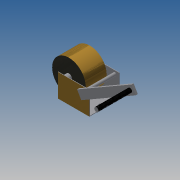
# Autodesk Inventor part: winch
Saved by Autodesk Inventor 2013 SP2 (Build 170200200, 200)
## iProperties
Created: 2013-12-16
Part Number: winch
Material: Generic
Document SubType Name: Modeling
Designer: Dave
Density: 1 g/cm^3
Author: Dave
Autodesk Inventor part; units mm, degrees
ref_plane "YZ Plane" through (0, 0, 0) normal (1, 0, 0) x (0, 1, 0)
ref_plane "XZ Plane" through (0, 0, 0) normal (0, 1, 0) x (-1, 0, 0)
ref_plane "XY Plane" through (0, 0, 0) normal (0, 0, 1) x (1, 0, 0)
sketch "Sketch1" plane through (0, 0, 0) normal (0, 0, 1) x (1, 0, 0)
  circle A0 centre (0, 0) radius 50.8
  dimension "d0" = 101.6
  constraints: 1 centre point, 1 coincident
  measures "d0" diameter of A0
extrude "Extrusion1" add sketch "Sketch1" along normal blind 63.5
sketch "Sketch2" plane through (0, 0, 63.5) normal (0, 0, 1) x (1, 0, 0)
  circle A0 centre (0, 0) radius 50.8 projected
  circle A1 centre (0, 0) radius 9.525
  dimension "d5" = 19.05
  constraints: 1 centre point, 1 coincident
  measures "d5" diameter of A1
extrude "Extrusion2" add sketch "Sketch2" along normal blind 15.875 and the other way blind 76.2 contours A1
sketch "Sketch3" plane through (0, 0, 79.375) normal (0, 0, 1) x (1, 0, 0)
  line L0 (-15.875, -55.5625) -> (79.375, -55.5625)
  line L1 (79.375, -55.5625) -> (79.375, 14.2875)
  line L2 (79.375, 14.2875) -> (-15.875, 14.2875)
  line L3 (-15.875, 14.2875) -> (-15.875, -55.5625)
  dimension "d11" = 95.25
  dimension "d13" = 69.85
  constraints: 8 end point, 2 parallel, 1 horizontal, 1 perpendicular
  measures "d11" distance of L0.start L0.end
  measures "d13" distance of L2.end L0.start
extrude "Extrusion3" add sketch "Sketch3" along normal blind 1.524
sketch "Sketch4" plane through (0, 0, 79.375) normal (0, 0, -1) x (-1, 0, 0)
  line L0 (15.875, -55.5625) -> (-79.375, -55.5625) projected
  line L1 (15.875, 14.2875) -> (15.875, -55.5625) projected
  line L2 (-79.375, -55.5625) -> (15.875, -55.5625)
  line L3 (15.875, -55.5625) -> (15.875, -54.0385)
  line L4 (15.875, -54.0385) -> (-79.375, -54.0385)
  line L5 (-79.375, -54.0385) -> (-79.375, -55.5625)
  point P0 (-79.375, 14.2875)
  dimension "d16" = 1.524
  dimension "d47" = 69.85
  dimension "d48" = 95.25
  constraints: 8 end point, 2 parallel, 1 horizontal, 1 perpendicular, 1 point on line
  measures "d16" distance of L4.end L0.end
  measures "d47" distance of L0.end point (-79.375, 14.288)
  measures "d48" distance of point (-79.375, 14.288) L1.start
extrude "Extrusion4" add sketch "Sketch4" along normal blind 88.9
sketch "Sketch5" plane through (0, 0, -9.525) normal (0, 0, -1) x (-1, 0, 0)
  line L0 (-79.375, -55.5625) -> (15.875, -55.5625)
  line L1 (15.875, -55.5625) -> (15.875, 14.2875)
  line L2 (15.875, 14.2875) -> (-79.375, 14.2875)
  line L3 (-79.375, 14.2875) -> (-79.375, -55.5625)
  point P0 (0, 0)
  constraints: 8 end point, 2 parallel, 1 horizontal, 1 perpendicular
extrude "Extrusion5" add sketch "Sketch5" along normal blind 1.524
sketch "Sketch6" plane through (0, 0, 80.899) normal (0, 0, 1) x (1, 0, 0)
  circle A0 centre (66.2655, 4.5181) radius 4.7625
  point P0 (0, 0)
  dimension "d21" = 9.525
  constraints: 1 centre point
  measures "d21" diameter of A0
extrude "Extrusion6" add sketch "Sketch6" along normal blind 12.7 and the other way blind 95.25
sketch "Sketch7" plane through (66.2655, 4.5181, 93.599) normal (0, 0, 1) x (1, 0, 0)
  line L0 (-5.1033, 11.8715) -> (159.8746, 107.1215)
  line L1 (159.8746, 107.1215) -> (172.5746, 85.1244)
  line L2 (172.5746, 85.1244) -> (7.5967, -10.1256)
  line L3 (7.5967, -10.1256) -> (-5.1033, 11.8715)
  line L4 (0, 0) -> (168.275, 0) construction
  point P0 (-66.2655, -4.5181)
  dimension "d29" = 25.4
  dimension "d30" = 190.5
  dimension "d40" = 30
  constraints: 10 end point, 2 parallel, 1 horizontal, 1 perpendicular
  measures "d29" distance of L2.end L0.start
  measures "d30" distance of L1.end L2.end
  measures "d40" angle of L4 L2
extrude "Extrusion7" add sketch "Sketch7" along normal blind 6.35
sketch "Sketch8" plane through (66.2655, 4.5181, 99.949) normal (0, 0, 1) x (1, 0, 0)
  line L0 (172.5746, 85.1244) -> (159.8746, 107.1215) projected
  circle A0 centre (155.226, 89.773) radius 6.35
  point P0 (-66.2655, -4.5181)
  dimension "d43" = 12.7
  dimension "d44" = 12.7
  constraints: 1 centre point
  measures "d43" diameter of A0
  measures "d44" distance from line of A0.centre L0
extrude "Extrusion8" add sketch "Sketch8" along normal blind 101.6
sketch "Sketch9" plane through (-15.875, -55.5625, 80.899) normal (0, -1, 0) x (1, 0, 0)
  line L0 (0, 0) -> (0, -91.948) projected
  line L1 (95.25, -91.948) -> (0, -91.948) projected
  circle A0 centre (12.7, -45.974) radius 4.7625
  circle A1 centre (82.55, -45.974) radius 4.7625
  point P0 (15.875, -80.899)
  dimension "d49" = 91.948
  dimension "d50" = 95.25
  dimension "d51" = 9.525
  dimension "d52" = 12.7
  dimension "d55" = 69.85
  constraints: 2 centre point, 1 horizontal, 2 other
  measures "d49" distance of L0.start L0.end
  measures "d50" distance of L1.start L0.end
  measures "d51" diameter of A0
  measures "d52" distance from line of A0.centre L0
  measures "d55" distance of A0.centre A1.centre
hole "Hole1" at (66.675, -55.5625, 34.925) at (-3.175, -55.5625, 34.925) direction (0, 1, 0) diameter 9.525 depth 2.54 tip angle 118
body "Solid1"
